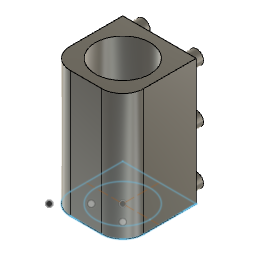
Versatip-holder v2 (Autodesk Fusion 360 design; units mm, degrees)
Autodesk Fusion 360 part; units mm, degrees
note: some values were not read from the file. Set by a fixed rule: which sketch regions a step uses.
sketch "Sketch1" plane through (0, 0, 0) normal (0, 0, 1) x (1, 0, 0)
  line L0 (12.5427, 32.7282) -> (47.5427, 32.7282)
  line L1 (47.5427, 32.7282) -> (47.5427, 7.7282)
  line L2 (37.5427, -2.2718) -> (22.5427, -2.2718)
  line L3 (12.5427, 7.7282) -> (12.5427, 32.7282)
  line L4 (47.5427, 15.2282) -> (12.5427, 15.2282) construction
  line L5 (30.0427, 32.7282) -> (30.0427, 15.2282) construction
  circle A0 centre (30.0427, 15.2282) radius 13
  arc A1 (12.5427, 7.7282) -> (22.5427, -2.2718) centre (22.5427, 7.7282) ccw
  arc A2 (37.5427, -2.2718) -> (47.5427, 7.7282) centre (37.5427, 7.7282) ccw
  point P0 (12.5427, -2.2718)
  dimension "d1" = 35
  dimension "d2" = 35
  dimension "d4" = 26
  dimension "d21" = 10
  constraint horizontal L0
  constraint vertical L1
  constraint horizontal L2
  constraint vertical L3
  constraint midpoint L0 L5.start
  constraint midpoint L4 L5.end
  constraint coincident L5.end A0.centre
  constraint coincident L3 L4.end
  constraint coincident P0 L2
  constraint coincident P0 L3
  constraint tangent L2 A1
  constraint tangent L3 A1
  constraint coincident L1 L4.start
  constraint tangent L1 A2
  constraint tangent L2 A2
  constraint equal A1 A2
  measures "d1" distance of L0.start L0.end
  measures "d2" distance of L0.start P0
  measures "d4" diameter of A0
  measures "d21" radius of A1
extrude "Extrude2" add sketch "Sketch1" along normal blind 20 makes body 1
extrude "Extrude1" add sketch "Sketch1" along normal blind 2 separate body contours L0 L1 L2 L3 A1 A2 | A0 makes body 2
combine "Combine1" operation add target body 1 tool bodies 2
extrude "Extrude3" add 1 faces at (25.9943, 15.2712, 2) along direction (0, 0, 1) blind 3 on bodies 1 bodies 1
extrude "Extrude4" add 1 faces at (45.9943, 19.2074, 20) along direction (0, 0, 1) blind 40 on bodies 1 bodies 1
sketch "Sketch2" plane through (0, 32.7282, 0) normal (0, 1, 0) x (-1, 0, 0)
  line L0 (-12.5427, 0) -> (-12.5427, 60)
  line L1 (-12.5427, 60) -> (-47.5427, 60)
  line L2 (-47.5427, 60) -> (-47.5427, 0)
  line L3 (-47.5427, 0) -> (-12.5427, 0)
  line L4 (-47.5427, 60) -> (-12.5427, 60)
  line L5 (-12.5427, 60) -> (-12.5427, 0)
  line L6 (-12.5427, 0) -> (-47.5427, 0)
  line L7 (-47.5427, 0) -> (-47.5427, 60)
  circle A0 centre (-42.7427, 5) radius 3.25
  circle A1 centre (-17.3427, 5) radius 3.25
  circle A2 centre (-42.7427, 30.4) radius 3.25
  circle A3 centre (-17.3427, 30.4) radius 3.25
  circle A4 centre (-42.7427, 55.8) radius 3.25
  circle A5 centre (-17.3427, 55.8) radius 3.25
  dimension "d15" = 6.5
  dimension "d16" = 4.8
  dimension "d19" = 25.4
  dimension "d20" = 25.4
  dimension "d22" = 5
  constraint horizontal L4
  constraint vertical L5
  constraint horizontal L6
  constraint vertical L7
  constraint coincident L0.start L3.end
  constraint coincident L1.end L2.start
  measures "d15" diameter of A0
  measures "d16" distance of L7 A0.centre
  measures "d22" distance of L6 A0.centre
extrude "Extrude5" add sketch "Sketch2" along normal blind 5 contours A0 | A1 | A2 | A3 | A4 | A5 bodies 1
equation "PegWidth = 6.5 mm"
equation "HoleDistance = 25.4 mm"
equation "d15 = PegWidth"
equation "d16 = ( 35 mm - HoleDistance ) / 2"
equation "d20 = HoleDistance"
